Autodesk Fusion 360 part; units mm, degrees
note: some values were not read from the file. Set by a fixed rule: which face or edge a step refers to.
(part 6 of 13)
sketch "Sketch1" plane through (0, 0, 0) normal (0, 0, 1) x (1, 0, 0)
  line L0 (0, 0) -> (25, 0)
  line L1 (25, 0) -> (25, 103)
  line L2 (25, 103) -> (0, 103)
  line L3 (0, 103) -> (0, 0)
  line L4 (0, 0) -> (2.25, 0)
  line L5 (0, 5) -> (25, 5)
  line L6 (0, 98) -> (25, 98)
  line L7 (0, 98) -> (7, 98)
  line L8 (7, 98) -> (7, 103)
  line L9 (7, 103) -> (0, 103)
  line L10 (0, 103) -> (0, 98)
  line L11 (7, 5) -> (0, 5)
  line L12 (0, 5) -> (0, 0)
  line L13 (0, 0) -> (7, 0)
  line L14 (7, 0) -> (7, 5)
  line L15 (10, 5) -> (17, 5)
  line L16 (17, 5) -> (17, 0)
  line L17 (17, 0) -> (10, 0)
  line L18 (10, 0) -> (10, 5)
  line L19 (10, 103) -> (17, 103)
  line L20 (17, 103) -> (17, 98)
  line L21 (17, 98) -> (10, 98)
  line L22 (10, 98) -> (10, 103)
  point P0 (25, 51.5)
  point P1 (25, 51.5)
  dimension "d1" = 25
  dimension "d2" = 103
  constraint horizontal L0
  constraint vertical L1
  constraint horizontal L2
  constraint vertical L3
  constraint coincident L0.start L3.end
  constraint coincident L0 L4.end
  constraint coincident L3 L5.start
  constraint coincident L1 L5.end
  constraint perpendicular L1 L5
  constraint coincident L3 L6.start
  constraint coincident L1 L6.end
  constraint perpendicular L1 L6
  constraint midpoint L1 P1
  constraint coincident P1 P0
  constraint horizontal L7
  constraint vertical L8
  constraint horizontal L9
  constraint vertical L10
  constraint horizontal L11
  constraint vertical L12
  constraint horizontal L13
  constraint vertical L14
  constraint coincident L5 L11.start
  constraint horizontal L15
  constraint vertical L16
  constraint horizontal L17
  constraint vertical L18
  constraint coincident L0 L16.end
  constraint coincident L5 L15.start
  constraint horizontal L19
  constraint vertical L20
  constraint horizontal L21
  constraint vertical L22
  constraint coincident L6 L20.end
  constraint coincident L2 L19.start
  measures "d1" distance of L0.start L0.end
  measures "d2" distance of L0.start L2.end
extrude "Extrude1" add sketch "Sketch1" along normal blind 2.5 contours L0 L3 L4 L5 L11 L12 L13 L14 | L1 L3 L5 L6 L7 L11 L15 L21 | L2 L3 L6 L7 L8 L9 L10 | L0 L5 L15 L16 L17 L18 | L2 L6 L19 L20 L21 L22 makes body 1
copy_body "CopyPasteBodies1" bodies 1 makes body 2
move_body "Move1" bodies 2 to x (1, 0, 0) y (0, 1, 0) z (0, 0, 1) at (37, 0, 0)
copy_body "Body->Comp1" bodies 1 removing the originals makes body 3 in component "Component"
copy_body "Body->Comp2" bodies 2 removing the originals makes body 4 in component "Component'"
component "Component" placed x (1, 0, 0) y (0, 1, 0) z (0, 0, 1) at (0, 0, 0)
component "Component'" placed x (1, 0, 0) y (0, 1, 0) z (0, 0, 1) at (0, 0, 0)

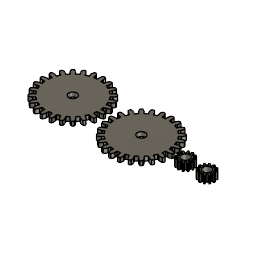
design "card-shuffler-middle-gears"
part number: 2026-08-17-02-18-25-515
part number: 2026-08-17-02-37-57-610
part number: 2026-08-17-02-39-26-180
Autodesk Fusion 360 part; units mm, degrees
sketch "Sketch1" plane through (0, 0, 0) normal (0, 0, 1) x (1, 0, 0) in component "Component"
  spline S0 degree 5 poles (4.55639, -0.625578) (4.556431, -0.625583) (4.556519, -0.625594) (4.556664, -0.625612) (4.556887, -0.625638) (4.557214, -0.625675) (4.557589, -0.625717) (4.558012, -0.625763) (4.558483, -0.625812) (4.559001, -0.625865) (4.559566, -0.625921) (4.560177, -0.62598) (4.560835, -0.62604) (4.561539, -0.626103) (4.562289, -0.626167) (4.563084, -0.626233) (4.563925, -0.626299) (4.564811, -0.626366) (4.565742, -0.626434) (4.566718, -0.626502) (4.567738, -0.62657) (4.568802, -0.626637) (4.569909, -0.626704) (4.571061, -0.626769) (4.572255, -0.626834) (4.573493, -0.626896) (4.574774, -0.626957) (4.576097, -0.627016) (4.577463, -0.627072) (4.578871, -0.627126) (4.580321, -0.627176) (4.581812, -0.627224) (4.583345, -0.627268) (4.584919, -0.627308) (4.586534, -0.627345) (4.58819, -0.627377) (4.589886, -0.627405) (4.591623, -0.627428) (4.5934, -0.627446) (4.595217, -0.627459) (4.597073, -0.627467) (4.598968, -0.627469) (4.600903, -0.627465) (4.602877, -0.627456) (4.60489, -0.627439) (4.606941, -0.627417) (4.60903, -0.627387) (4.611158, -0.627351) (4.613323, -0.627308) (4.615527, -0.627257) (4.617767, -0.627198) (4.620045, -0.627132) (4.62236, -0.627058) (4.624712, -0.626975) (4.6271, -0.626884) (4.629525, -0.626785) (4.631986, -0.626676) (4.634484, -0.626559) (4.637017, -0.626432) (4.639585, -0.626296) (4.642189, -0.626151) (4.644828, -0.625996) (4.647503, -0.62583) (4.650212, -0.625655) (4.652956, -0.625469) (4.655734, -0.625273) (4.658546, -0.625066) (4.661393, -0.624848) (4.664273, -0.624619) (4.667187, -0.624379) (4.670135, -0.624128) (4.673116, -0.623865) (4.67613, -0.62359) (4.679177, -0.623304) (4.682256, -0.623005) (4.685368, -0.622694) (4.688513, -0.622371) (4.691689, -0.622035) (4.694898, -0.621687) (4.698138, -0.621325) (4.70141, -0.620951) (4.704714, -0.620563) (4.708048, -0.620163) (4.711414, -0.619748) (4.714811, -0.61932) (4.718238, -0.618879) (4.721696, -0.618423) (4.725184, -0.617953) (4.728702, -0.61747) (4.732251, -0.616971) (4.735829, -0.616459) (4.739437, -0.615931) (4.743074, -0.615389) (4.74674, -0.614832) (4.750436, -0.61426) (4.754161, -0.613673) (4.757914, -0.613071) (4.761696, -0.612453) (4.765506, -0.611819) (4.769345, -0.61117) (4.773212, -0.610505) (4.777106, -0.609824) (4.781029, -0.609127) (4.784979, -0.608414) (4.788956, -0.607684) (4.792961, -0.606938) (4.796992, -0.606176) (4.801051, -0.605396) (4.805136, -0.6046) (4.809248, -0.603787) (4.813386, -0.602957) (4.817551, -0.60211) (4.821742, -0.601246) (4.825958, -0.600364) (4.830201, -0.599464) (4.834469, -0.598547) (4.838762, -0.597613) (4.843081, -0.59666) (4.847425, -0.59569) (4.851793, -0.594701) (4.856187, -0.593695) (4.860605, -0.59267) (4.865048, -0.591627) (4.869515, -0.590565) (4.874006, -0.589485) (4.878521, -0.588386) (4.88306, -0.587269) (4.887623, -0.586132) (4.892209, -0.584977) (4.896819, -0.583802) (4.901452, -0.582609) (4.906108, -0.581396) (4.910787, -0.580163) (4.915489, -0.578912) (4.920213, -0.577641) (4.92496, -0.57635) (4.929729, -0.57504) (4.93452, -0.573709) (4.939334, -0.572359) (4.944169, -0.570989) (4.949026, -0.569599) (4.953904, -0.568189) (4.958804, -0.566758) (4.963725, -0.565307) (4.968668, -0.563836) (4.973631, -0.562344) (4.978615, -0.560832) (4.98362, -0.559299) (4.988645, -0.557746) (4.993691, -0.556171) (4.998756, -0.554576) (5.003842, -0.55296) (5.008948, -0.551323) (5.014074, -0.549664) (5.01922, -0.547985) (5.024384, -0.546284) (5.029569, -0.544562) (5.034772, -0.542818) (5.039995, -0.541053) (5.045236, -0.539267) (5.050497, -0.537458) (5.055776, -0.535628) (5.061073, -0.533777) (5.066389, -0.531903) (5.071723, -0.530008) (5.077076, -0.528091) (5.082446, -0.526151) (5.087834, -0.52419) (5.093239, -0.522206) (5.098663, -0.5202) (5.104103, -0.518172) (5.109561, -0.516122) (5.115036, -0.514049) (5.120528, -0.511953) (5.126037, -0.509835) (5.131563, -0.507695) (5.137105, -0.505532) (5.142663, -0.503346) (5.148238, -0.501137) (5.153829, -0.498906) (5.159436, -0.496651) (5.165059, -0.494374) (5.170698, -0.492073) (5.176352, -0.48975) (5.182022, -0.487404) (5.187708, -0.485034) (5.193408, -0.482641) (5.199124, -0.480225) (5.204854, -0.477785) (5.210599, -0.475322) (5.21636, -0.472836) (5.222134, -0.470326) (5.227923, -0.467793) (5.233727, -0.465236) (5.239544, -0.462655) (5.245376, -0.460051) (5.251221, -0.457423) (5.257081, -0.454771) (5.262954, -0.452096) (5.26884, -0.449396) (5.27474, -0.446673) (5.280653, -0.443925) (5.28658, -0.441154) (5.292519, -0.438359) (5.298471, -0.435539) (5.304436, -0.432696) (5.310414, -0.429828) (5.316404, -0.426936) (5.322407, -0.42402) (5.328422, -0.421079) (5.334448, -0.418115) (5.340487, -0.415125) (5.346538, -0.412112) (5.352601, -0.409074) (5.358675, -0.406011) (5.364761, -0.402924) (5.370858, -0.399812) (5.376966, -0.396676) (5.383086, -0.393515) (5.389216, -0.39033) (5.395357, -0.387119) (5.40151, -0.383884) (5.407672, -0.380625) (5.413846, -0.37734) (5.420029, -0.374031) (5.426223, -0.370696) (5.432428, -0.367337) (5.438642, -0.363953) (5.444866, -0.360544) (5.4511, -0.35711) (5.457343, -0.353651) (5.463597, -0.350166) (5.469859, -0.346657) (5.476131, -0.343123) (5.482412, -0.339563) (5.488702, -0.335979) (5.495001, -0.332369) (5.501309, -0.328733) (5.507626, -0.325073) (5.513951, -0.321387) (5.520284, -0.317676) (5.525358, -0.314687) (5.529167, -0.312434) (5.531709, -0.310927) (5.53298, -0.310172) knots 0 0 0 0 0 0 0.00416667 0.00833333 0.0125 0.01666667 0.02083333 0.025 0.02916667 0.03333333 0.0375 0.04166667 0.04583333 0.05 0.05416667 0.05833333 0.0625 0.06666667 0.07083333 0.075 0.07916667 0.08333333 0.0875 0.09166667 0.09583333 0.1 0.10416667 0.10833333 0.1125 0.11666667 0.12083333 0.125 0.12916667 0.13333333 0.1375 0.14166667 0.14583333 0.15 0.15416667 0.15833333 0.1625 0.16666667 0.17083333 0.175 0.17916667 0.18333333 0.1875 0.19166667 0.19583333 0.2 0.20416667 0.20833333 0.2125 0.21666667 0.22083333 0.225 0.22916667 0.23333333 0.2375 0.24166667 0.24583333 0.25 0.25416667 0.25833333 0.2625 0.26666667 0.27083333 0.275 0.27916667 0.28333333 0.2875 0.29166667 0.29583333 0.3 0.30416667 0.30833333 0.3125 0.31666667 0.32083333 0.325 0.32916667 0.33333333 0.3375 0.34166667 0.34583333 0.35 0.35416667 0.35833333 0.3625 0.36666667 0.37083333 0.375 0.37916667 0.38333333 0.3875 0.39166667 0.39583333 0.4 0.40416667 0.40833333 0.4125 0.41666667 0.42083333 0.425 0.42916667 0.43333333 0.4375 0.44166667 0.44583333 0.45 0.45416667 0.45833333 0.4625 0.46666667 0.47083333 0.475 0.47916667 0.48333333 0.4875 0.49166667 0.49583333 0.5 0.50416667 0.50833333 0.5125 0.51666667 0.52083333 0.525 0.52916667 0.53333333 0.5375 0.54166667 0.54583333 0.55 0.55416667 0.55833333 0.5625 0.56666667 0.57083333 0.575 0.57916667 0.58333333 0.5875 0.59166667 0.59583333 0.6 0.60416667 0.60833333 0.6125 0.61666667 0.62083333 0.625 0.62916667 0.63333333 0.6375 0.64166667 0.64583333 0.65 0.65416667 0.65833333 0.6625 0.66666667 0.67083333 0.675 0.67916667 0.68333333 0.6875 0.69166667 0.69583333 0.7 0.70416667 0.70833333 0.7125 0.71666667 0.72083333 0.725 0.72916667 0.73333333 0.7375 0.74166667 0.74583333 0.75 0.75416667 0.75833333 0.7625 0.76666667 0.77083333 0.775 0.77916667 0.78333333 0.7875 0.79166667 0.79583333 0.8 0.80416667 0.80833333 0.8125 0.81666667 0.82083333 0.825 0.82916667 0.83333333 0.8375 0.84166667 0.84583333 0.85 0.85416667 0.85833333 0.8625 0.86666667 0.87083333 0.875 0.87916667 0.88333333 0.8875 0.89166667 0.89583333 0.9 0.90416667 0.90833333 0.9125 0.91666667 0.92083333 0.925 0.92916667 0.93333333 0.9375 0.94166667 0.94583333 0.95 0.95416667 0.95833333 0.9625 0.96666667 0.97083333 0.975 0.97916667 0.98333333 0.9875 0.99166667 0.99583333 1 1 1 1 1 1
  spline S1 degree 5 poles (4.55639, 0.625578) (4.556431, 0.625583) (4.556519, 0.625594) (4.556664, 0.625612) (4.556887, 0.625638) (4.557214, 0.625675) (4.557589, 0.625717) (4.558012, 0.625763) (4.558483, 0.625812) (4.559001, 0.625865) (4.559566, 0.625921) (4.560177, 0.62598) (4.560835, 0.62604) (4.561539, 0.626103) (4.562289, 0.626167) (4.563084, 0.626233) (4.563925, 0.626299) (4.564811, 0.626366) (4.565742, 0.626434) (4.566718, 0.626502) (4.567738, 0.62657) (4.568802, 0.626637) (4.569909, 0.626704) (4.571061, 0.626769) (4.572255, 0.626834) (4.573493, 0.626896) (4.574774, 0.626957) (4.576097, 0.627016) (4.577463, 0.627072) (4.578871, 0.627126) (4.580321, 0.627176) (4.581812, 0.627224) (4.583345, 0.627268) (4.584919, 0.627308) (4.586534, 0.627345) (4.58819, 0.627377) (4.589886, 0.627405) (4.591623, 0.627428) (4.5934, 0.627446) (4.595217, 0.627459) (4.597073, 0.627467) (4.598968, 0.627469) (4.600903, 0.627465) (4.602877, 0.627456) (4.60489, 0.627439) (4.606941, 0.627417) (4.60903, 0.627387) (4.611158, 0.627351) (4.613323, 0.627308) (4.615527, 0.627257) (4.617767, 0.627198) (4.620045, 0.627132) (4.62236, 0.627058) (4.624712, 0.626975) (4.6271, 0.626884) (4.629525, 0.626785) (4.631986, 0.626676) (4.634484, 0.626559) (4.637017, 0.626432) (4.639585, 0.626296) (4.642189, 0.626151) (4.644828, 0.625996) (4.647503, 0.62583) (4.650212, 0.625655) (4.652956, 0.625469) (4.655734, 0.625273) (4.658546, 0.625066) (4.661393, 0.624848) (4.664273, 0.624619) (4.667187, 0.624379) (4.670135, 0.624128) (4.673116, 0.623865) (4.67613, 0.62359) (4.679177, 0.623304) (4.682256, 0.623005) (4.685368, 0.622694) (4.688513, 0.622371) (4.691689, 0.622035) (4.694898, 0.621687) (4.698138, 0.621325) (4.70141, 0.620951) (4.704714, 0.620563) (4.708048, 0.620163) (4.711414, 0.619748) (4.714811, 0.61932) (4.718238, 0.618879) (4.721696, 0.618423) (4.725184, 0.617953) (4.728702, 0.61747) (4.732251, 0.616971) (4.735829, 0.616459) (4.739437, 0.615931) (4.743074, 0.615389) (4.74674, 0.614832) (4.750436, 0.61426) (4.754161, 0.613673) (4.757914, 0.613071) (4.761696, 0.612453) (4.765506, 0.611819) (4.769345, 0.61117) (4.773212, 0.610505) (4.777106, 0.609824) (4.781029, 0.609127) (4.784979, 0.608414) (4.788956, 0.607684) (4.792961, 0.606938) (4.796992, 0.606176) (4.801051, 0.605396) (4.805136, 0.6046) (4.809248, 0.603787) (4.813386, 0.602957) (4.817551, 0.60211) (4.821742, 0.601246) (4.825958, 0.600364) (4.830201, 0.599464) (4.834469, 0.598547) (4.838762, 0.597613) (4.843081, 0.59666) (4.847425, 0.59569) (4.851793, 0.594701) (4.856187, 0.593695) (4.860605, 0.59267) (4.865048, 0.591627) (4.869515, 0.590565) (4.874006, 0.589485) (4.878521, 0.588386) (4.88306, 0.587269) (4.887623, 0.586132) (4.892209, 0.584977) (4.896819, 0.583802) (4.901452, 0.582609) (4.906108, 0.581396) (4.910787, 0.580163) (4.915489, 0.578912) (4.920213, 0.577641) (4.92496, 0.57635) (4.929729, 0.57504) (4.93452, 0.573709) (4.939334, 0.572359) (4.944169, 0.570989) (4.949026, 0.569599) (4.953904, 0.568189) (4.958804, 0.566758) (4.963725, 0.565307) (4.968668, 0.563836) (4.973631, 0.562344) (4.978615, 0.560832) (4.98362, 0.559299) (4.988645, 0.557746) (4.993691, 0.556171) (4.998756, 0.554576) (5.003842, 0.55296) (5.008948, 0.551323) (5.014074, 0.549664) (5.01922, 0.547985) (5.024384, 0.546284) (5.029569, 0.544562) (5.034772, 0.542818) (5.039995, 0.541053) (5.045236, 0.539267) (5.050497, 0.537458) (5.055776, 0.535628) (5.061073, 0.533777) (5.066389, 0.531903) (5.071723, 0.530008) (5.077076, 0.528091) (5.082446, 0.526151) (5.087834, 0.52419) (5.093239, 0.522206) (5.098663, 0.5202) (5.104103, 0.518172) (5.109561, 0.516122) (5.115036, 0.514049) (5.120528, 0.511953) (5.126037, 0.509835) (5.131563, 0.507695) (5.137105, 0.505532) (5.142663, 0.503346) (5.148238, 0.501137) (5.153829, 0.498906) (5.159436, 0.496651) (5.165059, 0.494374) (5.170698, 0.492073) (5.176352, 0.48975) (5.182022, 0.487404) (5.187708, 0.485034) (5.193408, 0.482641) (5.199124, 0.480225) (5.204854, 0.477785) (5.210599, 0.475322) (5.21636, 0.472836) (5.222134, 0.470326) (5.227923, 0.467793) (5.233727, 0.465236) (5.239544, 0.462655) (5.245376, 0.460051) (5.251221, 0.457423) (5.257081, 0.454771) (5.262954, 0.452096) (5.26884, 0.449396) (5.27474, 0.446673) (5.280653, 0.443925) (5.28658, 0.441154) (5.292519, 0.438359) (5.298471, 0.435539) (5.304436, 0.432696) (5.310414, 0.429828) (5.316404, 0.426936) (5.322407, 0.42402) (5.328422, 0.421079) (5.334448, 0.418115) (5.340487, 0.415125) (5.346538, 0.412112) (5.352601, 0.409074) (5.358675, 0.406011) (5.364761, 0.402924) (5.370858, 0.399812) (5.376966, 0.396676) (5.383086, 0.393515) (5.389216, 0.39033) (5.395357, 0.387119) (5.40151, 0.383884) (5.407672, 0.380625) (5.413846, 0.37734) (5.420029, 0.374031) (5.426223, 0.370696) (5.432428, 0.367337) (5.438642, 0.363953) (5.444866, 0.360544) (5.4511, 0.35711) (5.457343, 0.353651) (5.463597, 0.350166) (5.469859, 0.346657) (5.476131, 0.343123) (5.482412, 0.339563) (5.488702, 0.335979) (5.495001, 0.332369) (5.501309, 0.328733) (5.507626, 0.325073) (5.513951, 0.321387) (5.520284, 0.317676) (5.525358, 0.314687) (5.529167, 0.312434) (5.531709, 0.310927) (5.53298, 0.310172) knots 0 0 0 0 0 0 0.00416667 0.00833333 0.0125 0.01666667 0.02083333 0.025 0.02916667 0.03333333 0.0375 0.04166667 0.04583333 0.05 0.05416667 0.05833333 0.0625 0.06666667 0.07083333 0.075 0.07916667 0.08333333 0.0875 0.09166667 0.09583333 0.1 0.10416667 0.10833333 0.1125 0.11666667 0.12083333 0.125 0.12916667 0.13333333 0.1375 0.14166667 0.14583333 0.15 0.15416667 0.15833333 0.1625 0.16666667 0.17083333 0.175 0.17916667 0.18333333 0.1875 0.19166667 0.19583333 0.2 0.20416667 0.20833333 0.2125 0.21666667 0.22083333 0.225 0.22916667 0.23333333 0.2375 0.24166667 0.24583333 0.25 0.25416667 0.25833333 0.2625 0.26666667 0.27083333 0.275 0.27916667 0.28333333 0.2875 0.29166667 0.29583333 0.3 0.30416667 0.30833333 0.3125 0.31666667 0.32083333 0.325 0.32916667 0.33333333 0.3375 0.34166667 0.34583333 0.35 0.35416667 0.35833333 0.3625 0.36666667 0.37083333 0.375 0.37916667 0.38333333 0.3875 0.39166667 0.39583333 0.4 0.40416667 0.40833333 0.4125 0.41666667 0.42083333 0.425 0.42916667 0.43333333 0.4375 0.44166667 0.44583333 0.45 0.45416667 0.45833333 0.4625 0.46666667 0.47083333 0.475 0.47916667 0.48333333 0.4875 0.49166667 0.49583333 0.5 0.50416667 0.50833333 0.5125 0.51666667 0.52083333 0.525 0.52916667 0.53333333 0.5375 0.54166667 0.54583333 0.55 0.55416667 0.55833333 0.5625 0.56666667 0.57083333 0.575 0.57916667 0.58333333 0.5875 0.59166667 0.59583333 0.6 0.60416667 0.60833333 0.6125 0.61666667 0.62083333 0.625 0.62916667 0.63333333 0.6375 0.64166667 0.64583333 0.65 0.65416667 0.65833333 0.6625 0.66666667 0.67083333 0.675 0.67916667 0.68333333 0.6875 0.69166667 0.69583333 0.7 0.70416667 0.70833333 0.7125 0.71666667 0.72083333 0.725 0.72916667 0.73333333 0.7375 0.74166667 0.74583333 0.75 0.75416667 0.75833333 0.7625 0.76666667 0.77083333 0.775 0.77916667 0.78333333 0.7875 0.79166667 0.79583333 0.8 0.80416667 0.80833333 0.8125 0.81666667 0.82083333 0.825 0.82916667 0.83333333 0.8375 0.84166667 0.84583333 0.85 0.85416667 0.85833333 0.8625 0.86666667 0.87083333 0.875 0.87916667 0.88333333 0.8875 0.89166667 0.89583333 0.9 0.90416667 0.90833333 0.9125 0.91666667 0.92083333 0.925 0.92916667 0.93333333 0.9375 0.94166667 0.94583333 0.95 0.95416667 0.95833333 0.9625 0.96666667 0.97083333 0.975 0.97916667 0.98333333 0.9875 0.99166667 0.99583333 1 1 1 1 1 1
  spline S2 degree 5 poles (4.55596, -0.625523) (4.555978, -0.625525) (4.556012, -0.625529) (4.556063, -0.625536) (4.556132, -0.625545) (4.556218, -0.625556) (4.556287, -0.625564) (4.556338, -0.625571) (4.556373, -0.625575) (4.55639, -0.625578) knots 0 0 0 0 0 0 0.2 0.4 0.6 0.8 1 1 1 1 1 1
  spline S3 degree 5 poles (4.55596, 0.625523) (4.555978, 0.625525) (4.556012, 0.625529) (4.556063, 0.625536) (4.556132, 0.625545) (4.556218, 0.625556) (4.556287, 0.625564) (4.556338, 0.625571) (4.556373, 0.625575) (4.55639, 0.625578) knots 0 0 0 0 0 0 0.2 0.4 0.6 0.8 1 1 1 1 1 1
  line L0 (0, 0) -> (4.55596, -0.625523)
  line L1 (0, 0) -> (4.55596, 0.625523)
  arc A0 (5.53298, -0.310172) -> (5.53298, 0.310172) centre (0, 0) ccw
  point P0 (4.55768, -0.625727)
  point P1 (4.559834, -0.625946)
  point P2 (4.562853, -0.626213)
  point P3 (4.56674, -0.626503)
  point P4 (4.571494, -0.626792)
  point P5 (4.577117, -0.627057)
  point P6 (4.583608, -0.627274)
  point P7 (4.590968, -0.627418)
  point P8 (4.599194, -0.627467)
  point P9 (4.608287, -0.627397)
  point P10 (4.618244, -0.627183)
  point P11 (4.629062, -0.626802)
  point P12 (4.640739, -0.626231)
  point P13 (4.653272, -0.625445)
  point P14 (4.666656, -0.624422)
  point P15 (4.680887, -0.623137)
  point P16 (4.69596, -0.621567)
  point P17 (4.711871, -0.619689)
  point P18 (4.728613, -0.617479)
  point P19 (4.74618, -0.614915)
  point P20 (4.764565, -0.611974)
  point P21 (4.783761, -0.608632)
  point P22 (4.803761, -0.604867)
  point P23 (4.824556, -0.600655)
  point P24 (4.846137, -0.595976)
  point P25 (4.868496, -0.590805)
  point P26 (4.891623, -0.585122)
  point P27 (4.915508, -0.578903)
  point P28 (4.94014, -0.572128)
  point P29 (4.965509, -0.564774)
  point P30 (4.991603, -0.556821)
  point P31 (5.01841, -0.548246)
  point P32 (5.045918, -0.539029)
  point P33 (5.074114, -0.52915)
  point P34 (5.102985, -0.518586)
  point P35 (5.132518, -0.507319)
  point P36 (5.162698, -0.495328)
  point P37 (5.193511, -0.482593)
  point P38 (5.224943, -0.469095)
  point P39 (5.256977, -0.454814)
  point P40 (5.289598, -0.439731)
  point P41 (5.32279, -0.423829)
  point P42 (5.356536, -0.407087)
  point P43 (5.39082, -0.389488)
  point P44 (5.425624, -0.371015)
  point P45 (5.460931, -0.351649)
  point P46 (5.496722, -0.331374)
  point P47 (4.55768, 0.625727)
  point P48 (4.559834, 0.625946)
  point P49 (4.562853, 0.626213)
  point P50 (4.56674, 0.626503)
  point P51 (4.571494, 0.626792)
  point P52 (4.577117, 0.627057)
  point P53 (4.583608, 0.627274)
  point P54 (4.590968, 0.627418)
  point P55 (4.599194, 0.627467)
  point P56 (4.608287, 0.627397)
  point P57 (4.618244, 0.627183)
  point P58 (4.629062, 0.626802)
  point P59 (4.640739, 0.626231)
  point P60 (4.653272, 0.625445)
  point P61 (4.666656, 0.624422)
  point P62 (4.680887, 0.623137)
  point P63 (4.69596, 0.621567)
  point P64 (4.711871, 0.619689)
  point P65 (4.728613, 0.617479)
  point P66 (4.74618, 0.614915)
  point P67 (4.764565, 0.611974)
  point P68 (4.783761, 0.608632)
  point P69 (4.803761, 0.604867)
  point P70 (4.824556, 0.600655)
  point P71 (4.846137, 0.595976)
  point P72 (4.868496, 0.590805)
  point P73 (4.891623, 0.585122)
  point P74 (4.915508, 0.578903)
  point P75 (4.94014, 0.572128)
  point P76 (4.965509, 0.564774)
  point P77 (4.991603, 0.556821)
  point P78 (5.01841, 0.548246)
  point P79 (5.045918, 0.539029)
  point P80 (5.074114, 0.52915)
  point P81 (5.102985, 0.518586)
  point P82 (5.132518, 0.507319)
  point P83 (5.162698, 0.495328)
  point P84 (5.193511, 0.482593)
  point P85 (5.224943, 0.469095)
  point P86 (5.256977, 0.454814)
  point P87 (5.289598, 0.439731)
  point P88 (5.32279, 0.423829)
  point P89 (5.356536, 0.407087)
  point P90 (5.39082, 0.389488)
  point P91 (5.425624, 0.371015)
  point P92 (5.460931, 0.351649)
  point P93 (5.496722, 0.331374)
sketch "Sketch2" plane through (0, 0, 0) normal (0, 0, 1) x (1, 0, 0) in component "Component"
  circle A0 centre (0, 0) radius 3.760417
extrude "Extrude1" add sketch "Sketch2" along normal blind 5 contours A0 picked at (-1.408263, 1.026971) makes body 1 in component "Component"
extrude "Extrude2" add sketch "Sketch1" along normal blind 5 separate body contours S0 S1 L0 L1 A0 picked at (3.037593, 0) makes body 2 in component "Component"
pattern_circular "C-Pattern1" count 12 over 360 about axis through (0, 0, 1.75) along (0, 0, 1) of "Extrude2" makes body 3 at (1.419579, 0.57881, 1.666667) makes body 4 at (0.939987, 1.211054, 1.666667) makes body 5 at (0.208526, 1.518797, 1.666667) makes body 6 at (-0.57881, 1.419579, 1.666667) makes body 7 at (-1.419579, 0.57881, 1.666667) makes body 8 at (-1.518797, 0.208526, 1.666667) makes body 9 at (-1.419579, -0.57881, 1.666667) makes body 10 at (-0.939987, -1.211054, 1.666667) makes body 11 at (-0.208526, -1.518797, 1.666667) makes body 12 at (0.57881, -1.419579, 1.666667) makes body 13 at (1.211054, -0.939987, 1.666667) in component "Component"
combine "Combine1" operation add target body 1 tool bodies 2 3 4 5 6 7 8 9 10 11 12 13 in component "Component"
sketch "Sketch3" plane through (0, 0, 0) normal (0, 0, 1) x (1, 0, 0) in component "Component"
  line L0 (0, 0) -> (51.568365, 0) construction
  line L1 (51.568365, 0) -> (51.568365, 3) construction
  line L2 (51.568365, 3) -> (0, 3) construction
  line L3 (0, 3) -> (0, 0) construction
  constraint perpendicular L0 L1
  constraint parallel L0 L2
  constraint parallel L1 L3
sketch "Sketch1 (2)" plane through (0, 0, 0) normal (0, 0, 1) x (1, 0, 0) in component "Component'"
  spline S0 degree 5 poles (19.838391, -1.410784) (19.83851, -1.410792) (19.838764, -1.410808) (19.839192, -1.410833) (19.839856, -1.410871) (19.840843, -1.410923) (19.841984, -1.410981) (19.84328, -1.411043) (19.844726, -1.411108) (19.84632, -1.411176) (19.848058, -1.411245) (19.849938, -1.411314) (19.851959, -1.411383) (19.854118, -1.411451) (19.856413, -1.411516) (19.858843, -1.411579) (19.861405, -1.411638) (19.864098, -1.411693) (19.86692, -1.411744) (19.869868, -1.411788) (19.872941, -1.411827) (19.876138, -1.411858) (19.879457, -1.411882) (19.882895, -1.411898) (19.886453, -1.411905) (19.890128, -1.411903) (19.893918, -1.411891) (19.897823, -1.411869) (19.90184, -1.411836) (19.905969, -1.411791) (19.910209, -1.411734) (19.914557, -1.411665) (19.919012, -1.411583) (19.923574, -1.411488) (19.928241, -1.411379) (19.933012, -1.411256) (19.937885, -1.411117) (19.942861, -1.410964) (19.947936, -1.410795) (19.953111, -1.410611) (19.958385, -1.410409) (19.963755, -1.410191) (19.969222, -1.409956) (19.974784, -1.409704) (19.98044, -1.409433) (19.98619, -1.409145) (19.992032, -1.408837) (19.997965, -1.408511) (20.003989, -1.408165) (20.010102, -1.4078) (20.016304, -1.407415) (20.022593, -1.407009) (20.02897, -1.406583) (20.035433, -1.406137) (20.041981, -1.405668) (20.048613, -1.405179) (20.05533, -1.404668) (20.062129, -1.404134) (20.06901, -1.403579) (20.075973, -1.403) (20.083016, -1.402399) (20.090139, -1.401775) (20.097341, -1.401127) (20.104622, -1.400456) (20.111981, -1.399761) (20.119417, -1.399041) (20.126929, -1.398298) (20.134516, -1.397529) (20.142179, -1.396736) (20.149917, -1.395918) (20.157728, -1.395074) (20.165612, -1.394205) (20.173569, -1.39331) (20.181598, -1.392389) (20.189698, -1.391442) (20.197868, -1.390469) (20.206109, -1.389469) (20.21442, -1.388442) (20.222799, -1.387389) (20.231247, -1.386308) (20.239763, -1.385199) (20.248346, -1.384064) (20.256996, -1.3829) (20.265712, -1.381709) (20.274494, -1.380489) (20.283341, -1.379241) (20.292252, -1.377965) (20.301228, -1.37666) (20.310268, -1.375327) (20.31937, -1.373964) (20.328536, -1.372572) (20.337763, -1.371151) (20.347052, -1.369701) (20.356403, -1.368221) (20.365814, -1.366711) (20.375285, -1.365172) (20.384817, -1.363602) (20.394407, -1.362002) (20.404057, -1.360372) (20.413765, -1.358711) (20.423531, -1.35702) (20.433355, -1.355298) (20.443236, -1.353545) (20.453174, -1.351761) (20.463168, -1.349945) (20.473218, -1.348099) (20.483323, -1.346221) (20.493484, -1.344312) (20.503699, -1.342371) (20.513969, -1.340398) (20.524292, -1.338393) (20.534669, -1.336356) (20.545099, -1.334287) (20.555582, -1.332185) (20.566117, -1.330052) (20.576704, -1.327885) (20.587343, -1.325687) (20.598033, -1.323455) (20.608774, -1.321191) (20.619565, -1.318893) (20.630407, -1.316563) (20.641298, -1.314199) (20.652239, -1.311802) (20.663229, -1.309372) (20.674268, -1.306908) (20.685354, -1.304411) (20.69649, -1.30188) (20.707672, -1.299315) (20.718902, -1.296717) (20.73018, -1.294084) (20.741503, -1.291418) (20.752874, -1.288717) (20.76429, -1.285982) (20.775752, -1.283213) (20.78726, -1.280409) (20.798812, -1.277571) (20.81041, -1.274698) (20.822052, -1.271791) (20.833738, -1.268848) (20.845468, -1.265871) (20.857241, -1.262859) (20.869058, -1.259813) (20.880918, -1.256731) (20.892821, -1.253613) (20.904765, -1.250461) (20.916752, -1.247273) (20.928781, -1.24405) (20.940851, -1.240792) (20.952963, -1.237498) (20.965115, -1.234168) (20.977308, -1.230803) (20.989542, -1.227402) (21.001815, -1.223965) (21.014129, -1.220492) (21.026482, -1.216983) (21.038874, -1.213439) (21.051305, -1.209858) (21.063775, -1.206241) (21.076283, -1.202588) (21.08883, -1.198898) (21.101415, -1.195172) (21.114037, -1.19141) (21.126697, -1.187612) (21.139394, -1.183776) (21.152128, -1.179905) (21.164898, -1.175996) (21.177705, -1.172051) (21.190548, -1.168069) (21.203427, -1.164051) (21.216342, -1.159995) (21.229292, -1.155903) (21.242277, -1.151773) (21.255297, -1.147607) (21.268352, -1.143403) (21.281442, -1.139162) (21.294565, -1.134884) (21.307723, -1.130569) (21.320914, -1.126217) (21.334139, -1.121827) (21.347397, -1.1174) (21.360689, -1.112935) (21.374013, -1.108433) (21.387369, -1.103894) (21.400758, -1.099316) (21.41418, -1.094702) (21.427633, -1.090049) (21.441117, -1.085359) (21.454634, -1.080631) (21.468181, -1.075865) (21.48176, -1.071062) (21.495369, -1.06622) (21.509009, -1.061341) (21.52268, -1.056423) (21.53638, -1.051468) (21.550111, -1.046475) (21.563871, -1.041443) (21.577661, -1.036373) (21.59148, -1.031266) (21.605329, -1.02612) (21.619206, -1.020935) (21.633112, -1.015713) (21.647047, -1.010452) (21.66101, -1.005153) (21.675, -0.999815) (21.689019, -0.994439) (21.703066, -0.989025) (21.71714, -0.983572) (21.731241, -0.97808) (21.74537, -0.97255) (21.759525, -0.966982) (21.773707, -0.961375) (21.787916, -0.955729) (21.802151, -0.950044) (21.816412, -0.944321) (21.830699, -0.938559) (21.845012, -0.932758) (21.859351, -0.926919) (21.873715, -0.921041) (21.888104, -0.915123) (21.902518, -0.909167) (21.916957, -0.903173) (21.93142, -0.897139) (21.945908, -0.891066) (21.96042, -0.884954) (21.974957, -0.878803) (21.989517, -0.872613) (22.004101, -0.866384) (22.018708, -0.860116) (22.033339, -0.853809) (22.047993, -0.847463) (22.062671, -0.841078) (22.077371, -0.834653) (22.092094, -0.828189) (22.106839, -0.821687) (22.121606, -0.815144) (22.136396, -0.808563) (22.151207, -0.801942) (22.16604, -0.795282) (22.180895, -0.788583) (22.195771, -0.781844) (22.210669, -0.775066) (22.222604, -0.769612) (22.231565, -0.765504) (22.237543, -0.762757) (22.240534, -0.761382) knots 0 0 0 0 0 0 0.00416667 0.00833333 0.0125 0.01666667 0.02083333 0.025 0.02916667 0.03333333 0.0375 0.04166667 0.04583333 0.05 0.05416667 0.05833333 0.0625 0.06666667 0.07083333 0.075 0.07916667 0.08333333 0.0875 0.09166667 0.09583333 0.1 0.10416667 0.10833333 0.1125 0.11666667 0.12083333 0.125 0.12916667 0.13333333 0.1375 0.14166667 0.14583333 0.15 0.15416667 0.15833333 0.1625 0.16666667 0.17083333 0.175 0.17916667 0.18333333 0.1875 0.19166667 0.19583333 0.2 0.20416667 0.20833333 0.2125 0.21666667 0.22083333 0.225 0.22916667 0.23333333 0.2375 0.24166667 0.24583333 0.25 0.25416667 0.25833333 0.2625 0.26666667 0.27083333 0.275 0.27916667 0.28333333 0.2875 0.29166667 0.29583333 0.3 0.30416667 0.30833333 0.3125 0.31666667 0.32083333 0.325 0.32916667 0.33333333 0.3375 0.34166667 0.34583333 0.35 0.35416667 0.35833333 0.3625 0.36666667 0.37083333 0.375 0.37916667 0.38333333 0.3875 0.39166667 0.39583333 0.4 0.40416667 0.40833333 0.4125 0.41666667 0.42083333 0.425 0.42916667 0.43333333 0.4375 0.44166667 0.44583333 0.45 0.45416667 0.45833333 0.4625 0.46666667 0.47083333 0.475 0.47916667 0.48333333 0.4875 0.49166667 0.49583333 0.5 0.50416667 0.50833333 0.5125 0.51666667 0.52083333 0.525 0.52916667 0.53333333 0.5375 0.54166667 0.54583333 0.55 0.55416667 0.55833333 0.5625 0.56666667 0.57083333 0.575 0.57916667 0.58333333 0.5875 0.59166667 0.59583333 0.6 0.60416667 0.60833333 0.6125 0.61666667 0.62083333 0.625 0.62916667 0.63333333 0.6375 0.64166667 0.64583333 0.65 0.65416667 0.65833333 0.6625 0.66666667 0.67083333 0.675 0.67916667 0.68333333 0.6875 0.69166667 0.69583333 0.7 0.70416667 0.70833333 0.7125 0.71666667 0.72083333 0.725 0.72916667 0.73333333 0.7375 0.74166667 0.74583333 0.75 0.75416667 0.75833333 0.7625 0.76666667 0.77083333 0.775 0.77916667 0.78333333 0.7875 0.79166667 0.79583333 0.8 0.80416667 0.80833333 0.8125 0.81666667 0.82083333 0.825 0.82916667 0.83333333 0.8375 0.84166667 0.84583333 0.85 0.85416667 0.85833333 0.8625 0.86666667 0.87083333 0.875 0.87916667 0.88333333 0.8875 0.89166667 0.89583333 0.9 0.90416667 0.90833333 0.9125 0.91666667 0.92083333 0.925 0.92916667 0.93333333 0.9375 0.94166667 0.94583333 0.95 0.95416667 0.95833333 0.9625 0.96666667 0.97083333 0.975 0.97916667 0.98333333 0.9875 0.99166667 0.99583333 1 1 1 1 1 1
  spline S1 degree 5 poles (19.838391, 1.410784) (19.83851, 1.410792) (19.838764, 1.410808) (19.839192, 1.410833) (19.839856, 1.410871) (19.840843, 1.410923) (19.841984, 1.410981) (19.84328, 1.411043) (19.844726, 1.411108) (19.84632, 1.411176) (19.848058, 1.411245) (19.849938, 1.411314) (19.851959, 1.411383) (19.854118, 1.411451) (19.856413, 1.411516) (19.858843, 1.411579) (19.861405, 1.411638) (19.864098, 1.411693) (19.86692, 1.411744) (19.869868, 1.411788) (19.872941, 1.411827) (19.876138, 1.411858) (19.879457, 1.411882) (19.882895, 1.411898) (19.886453, 1.411905) (19.890128, 1.411903) (19.893918, 1.411891) (19.897823, 1.411869) (19.90184, 1.411836) (19.905969, 1.411791) (19.910209, 1.411734) (19.914557, 1.411665) (19.919012, 1.411583) (19.923574, 1.411488) (19.928241, 1.411379) (19.933012, 1.411256) (19.937885, 1.411117) (19.942861, 1.410964) (19.947936, 1.410795) (19.953111, 1.410611) (19.958385, 1.410409) (19.963755, 1.410191) (19.969222, 1.409956) (19.974784, 1.409704) (19.98044, 1.409433) (19.98619, 1.409145) (19.992032, 1.408837) (19.997965, 1.408511) (20.003989, 1.408165) (20.010102, 1.4078) (20.016304, 1.407415) (20.022593, 1.407009) (20.02897, 1.406583) (20.035433, 1.406137) (20.041981, 1.405668) (20.048613, 1.405179) (20.05533, 1.404668) (20.062129, 1.404134) (20.06901, 1.403579) (20.075973, 1.403) (20.083016, 1.402399) (20.090139, 1.401775) (20.097341, 1.401127) (20.104622, 1.400456) (20.111981, 1.399761) (20.119417, 1.399041) (20.126929, 1.398298) (20.134516, 1.397529) (20.142179, 1.396736) (20.149917, 1.395918) (20.157728, 1.395074) (20.165612, 1.394205) (20.173569, 1.39331) (20.181598, 1.392389) (20.189698, 1.391442) (20.197868, 1.390469) (20.206109, 1.389469) (20.21442, 1.388442) (20.222799, 1.387389) (20.231247, 1.386308) (20.239763, 1.385199) (20.248346, 1.384064) (20.256996, 1.3829) (20.265712, 1.381709) (20.274494, 1.380489) (20.283341, 1.379241) (20.292252, 1.377965) (20.301228, 1.37666) (20.310268, 1.375327) (20.31937, 1.373964) (20.328536, 1.372572) (20.337763, 1.371151) (20.347052, 1.369701) (20.356403, 1.368221) (20.365814, 1.366711) (20.375285, 1.365172) (20.384817, 1.363602) (20.394407, 1.362002) (20.404057, 1.360372) (20.413765, 1.358711) (20.423531, 1.35702) (20.433355, 1.355298) (20.443236, 1.353545) (20.453174, 1.351761) (20.463168, 1.349945) (20.473218, 1.348099) (20.483323, 1.346221) (20.493484, 1.344312) (20.503699, 1.342371) (20.513969, 1.340398) (20.524292, 1.338393) (20.534669, 1.336356) (20.545099, 1.334287) (20.555582, 1.332185) (20.566117, 1.330052) (20.576704, 1.327885) (20.587343, 1.325687) (20.598033, 1.323455) (20.608774, 1.321191) (20.619565, 1.318893) (20.630407, 1.316563) (20.641298, 1.314199) (20.652239, 1.311802) (20.663229, 1.309372) (20.674268, 1.306908) (20.685354, 1.304411) (20.69649, 1.30188) (20.707672, 1.299315) (20.718902, 1.296717) (20.73018, 1.294084) (20.741503, 1.291418) (20.752874, 1.288717) (20.76429, 1.285982) (20.775752, 1.283213) (20.78726, 1.280409) (20.798812, 1.277571) (20.81041, 1.274698) (20.822052, 1.271791) (20.833738, 1.268848) (20.845468, 1.265871) (20.857241, 1.262859) (20.869058, 1.259813) (20.880918, 1.256731) (20.892821, 1.253613) (20.904765, 1.250461) (20.916752, 1.247273) (20.928781, 1.24405) (20.940851, 1.240792) (20.952963, 1.237498) (20.965115, 1.234168) (20.977308, 1.230803) (20.989542, 1.227402) (21.001815, 1.223965) (21.014129, 1.220492) (21.026482, 1.216983) (21.038874, 1.213439) (21.051305, 1.209858) (21.063775, 1.206241) (21.076283, 1.202588) (21.08883, 1.198898) (21.101415, 1.195172) (21.114037, 1.19141) (21.126697, 1.187612) (21.139394, 1.183776) (21.152128, 1.179905) (21.164898, 1.175996) (21.177705, 1.172051) (21.190548, 1.168069) (21.203427, 1.164051) (21.216342, 1.159995) (21.229292, 1.155903) (21.242277, 1.151773) (21.255297, 1.147607) (21.268352, 1.143403) (21.281442, 1.139162) (21.294565, 1.134884) (21.307723, 1.130569) (21.320914, 1.126217) (21.334139, 1.121827) (21.347397, 1.1174) (21.360689, 1.112935) (21.374013, 1.108433) (21.387369, 1.103894) (21.400758, 1.099316) (21.41418, 1.094702) (21.427633, 1.090049) (21.441117, 1.085359) (21.454634, 1.080631) (21.468181, 1.075865) (21.48176, 1.071062) (21.495369, 1.06622) (21.509009, 1.061341) (21.52268, 1.056423) (21.53638, 1.051468) (21.550111, 1.046475) (21.563871, 1.041443) (21.577661, 1.036373) (21.59148, 1.031266) (21.605329, 1.02612) (21.619206, 1.020935) (21.633112, 1.015713) (21.647047, 1.010452) (21.66101, 1.005153) (21.675, 0.999815) (21.689019, 0.994439) (21.703066, 0.989025) (21.71714, 0.983572) (21.731241, 0.97808) (21.74537, 0.97255) (21.759525, 0.966982) (21.773707, 0.961375) (21.787916, 0.955729) (21.802151, 0.950044) (21.816412, 0.944321) (21.830699, 0.938559) (21.845012, 0.932758) (21.859351, 0.926919) (21.873715, 0.921041) (21.888104, 0.915123) (21.902518, 0.909167) (21.916957, 0.903173) (21.93142, 0.897139) (21.945908, 0.891066) (21.96042, 0.884954) (21.974957, 0.878803) (21.989517, 0.872613) (22.004101, 0.866384) (22.018708, 0.860116) (22.033339, 0.853809) (22.047993, 0.847463) (22.062671, 0.841078) (22.077371, 0.834653) (22.092094, 0.828189) (22.106839, 0.821687) (22.121606, 0.815144) (22.136396, 0.808563) (22.151207, 0.801942) (22.16604, 0.795282) (22.180895, 0.788583) (22.195771, 0.781844) (22.210669, 0.775066) (22.222604, 0.769612) (22.231565, 0.765504) (22.237543, 0.762757) (22.240534, 0.761382) knots 0 0 0 0 0 0 0.00416667 0.00833333 0.0125 0.01666667 0.02083333 0.025 0.02916667 0.03333333 0.0375 0.04166667 0.04583333 0.05 0.05416667 0.05833333 0.0625 0.06666667 0.07083333 0.075 0.07916667 0.08333333 0.0875 0.09166667 0.09583333 0.1 0.10416667 0.10833333 0.1125 0.11666667 0.12083333 0.125 0.12916667 0.13333333 0.1375 0.14166667 0.14583333 0.15 0.15416667 0.15833333 0.1625 0.16666667 0.17083333 0.175 0.17916667 0.18333333 0.1875 0.19166667 0.19583333 0.2 0.20416667 0.20833333 0.2125 0.21666667 0.22083333 0.225 0.22916667 0.23333333 0.2375 0.24166667 0.24583333 0.25 0.25416667 0.25833333 0.2625 0.26666667 0.27083333 0.275 0.27916667 0.28333333 0.2875 0.29166667 0.29583333 0.3 0.30416667 0.30833333 0.3125 0.31666667 0.32083333 0.325 0.32916667 0.33333333 0.3375 0.34166667 0.34583333 0.35 0.35416667 0.35833333 0.3625 0.36666667 0.37083333 0.375 0.37916667 0.38333333 0.3875 0.39166667 0.39583333 0.4 0.40416667 0.40833333 0.4125 0.41666667 0.42083333 0.425 0.42916667 0.43333333 0.4375 0.44166667 0.44583333 0.45 0.45416667 0.45833333 0.4625 0.46666667 0.47083333 0.475 0.47916667 0.48333333 0.4875 0.49166667 0.49583333 0.5 0.50416667 0.50833333 0.5125 0.51666667 0.52083333 0.525 0.52916667 0.53333333 0.5375 0.54166667 0.54583333 0.55 0.55416667 0.55833333 0.5625 0.56666667 0.57083333 0.575 0.57916667 0.58333333 0.5875 0.59166667 0.59583333 0.6 0.60416667 0.60833333 0.6125 0.61666667 0.62083333 0.625 0.62916667 0.63333333 0.6375 0.64166667 0.64583333 0.65 0.65416667 0.65833333 0.6625 0.66666667 0.67083333 0.675 0.67916667 0.68333333 0.6875 0.69166667 0.69583333 0.7 0.70416667 0.70833333 0.7125 0.71666667 0.72083333 0.725 0.72916667 0.73333333 0.7375 0.74166667 0.74583333 0.75 0.75416667 0.75833333 0.7625 0.76666667 0.77083333 0.775 0.77916667 0.78333333 0.7875 0.79166667 0.79583333 0.8 0.80416667 0.80833333 0.8125 0.81666667 0.82083333 0.825 0.82916667 0.83333333 0.8375 0.84166667 0.84583333 0.85 0.85416667 0.85833333 0.8625 0.86666667 0.87083333 0.875 0.87916667 0.88333333 0.8875 0.89166667 0.89583333 0.9 0.90416667 0.90833333 0.9125 0.91666667 0.92083333 0.925 0.92916667 0.93333333 0.9375 0.94166667 0.94583333 0.95 0.95416667 0.95833333 0.9625 0.96666667 0.97083333 0.975 0.97916667 0.98333333 0.9875 0.99166667 0.99583333 1 1 1 1 1 1
  spline S2 degree 5 poles (19.837349, -1.410717) (19.837391, -1.41072) (19.837474, -1.410725) (19.837599, -1.410733) (19.837766, -1.410744) (19.837974, -1.410758) (19.838141, -1.410768) (19.838266, -1.410776) (19.838349, -1.410782) (19.838391, -1.410784) knots 0 0 0 0 0 0 0.2 0.4 0.6 0.8 1 1 1 1 1 1
  spline S3 degree 5 poles (19.837349, 1.410717) (19.837391, 1.41072) (19.837474, 1.410725) (19.837599, 1.410733) (19.837766, 1.410744) (19.837974, 1.410758) (19.838141, 1.410768) (19.838266, 1.410776) (19.838349, 1.410782) (19.838391, 1.410784) knots 0 0 0 0 0 0 0.2 0.4 0.6 0.8 1 1 1 1 1 1
  line L0 (0, 0) -> (19.837349, -1.410717)
  line L1 (0, 0) -> (19.837349, 1.410717)
  arc A0 (22.240534, -0.761382) -> (22.240534, 0.761382) centre (0, 0) ccw
  point P0 (19.841518, -1.410957)
  point P1 (19.846734, -1.411192)
  point P2 (19.854038, -1.411447)
  point P3 (19.863432, -1.411679)
  point P4 (19.874916, -1.411845)
  point P5 (19.888489, -1.411903)
  point P6 (19.90415, -1.411809)
  point P7 (19.921897, -1.411522)
  point P8 (19.941728, -1.410997)
  point P9 (19.963639, -1.410193)
  point P10 (19.987626, -1.409067)
  point P11 (20.013686, -1.407576)
  point P12 (20.041812, -1.405677)
  point P13 (20.072, -1.403328)
  point P14 (20.104242, -1.400487)
  point P15 (20.138531, -1.397112)
  point P16 (20.17486, -1.393159)
  point P17 (20.213219, -1.388587)
  point P18 (20.253601, -1.383354)
  point P19 (20.295995, -1.377419)
  point P20 (20.340392, -1.370738)
  point P21 (20.386778, -1.363271)
  point P22 (20.435145, -1.354977)
  point P23 (20.485478, -1.345813)
  point P24 (20.537764, -1.335739)
  point P25 (20.591992, -1.324713)
  point P26 (20.648145, -1.312696)
  point P27 (20.70621, -1.299646)
  point P28 (20.76617, -1.285523)
  point P29 (20.828011, -1.270287)
  point P30 (20.891714, -1.253898)
  point P31 (20.957263, -1.236316)
  point P32 (21.024639, -1.217502)
  point P33 (21.093825, -1.197416)
  point P34 (21.1648, -1.17602)
  point P35 (21.237546, -1.153274)
  point P36 (21.312041, -1.129141)
  point P37 (21.388265, -1.103582)
  point P38 (21.466195, -1.076559)
  point P39 (21.545811, -1.048034)
  point P40 (21.627089, -1.017971)
  point P41 (21.710005, -0.986333)
  point P42 (21.794536, -0.953082)
  point P43 (21.880658, -0.918182)
  point P44 (21.968344, -0.881598)
  point P45 (22.05757, -0.843293)
  point P46 (22.148309, -0.803233)
  point P47 (19.841518, 1.410957)
  point P48 (19.846734, 1.411192)
  point P49 (19.854038, 1.411447)
  point P50 (19.863432, 1.411679)
  point P51 (19.874916, 1.411845)
  point P52 (19.888489, 1.411903)
  point P53 (19.90415, 1.411809)
  point P54 (19.921897, 1.411522)
  point P55 (19.941728, 1.410997)
  point P56 (19.963639, 1.410193)
  point P57 (19.987626, 1.409067)
  point P58 (20.013686, 1.407576)
  point P59 (20.041812, 1.405677)
  point P60 (20.072, 1.403328)
  point P61 (20.104242, 1.400487)
  point P62 (20.138531, 1.397112)
  point P63 (20.17486, 1.393159)
  point P64 (20.213219, 1.388587)
  point P65 (20.253601, 1.383354)
  point P66 (20.295995, 1.377419)
  point P67 (20.340392, 1.370738)
  point P68 (20.386778, 1.363271)
  point P69 (20.435145, 1.354977)
  point P70 (20.485478, 1.345813)
  point P71 (20.537764, 1.335739)
  point P72 (20.591992, 1.324713)
  point P73 (20.648145, 1.312696)
  point P74 (20.70621, 1.299646)
  point P75 (20.76617, 1.285523)
  point P76 (20.828011, 1.270287)
  point P77 (20.891714, 1.253898)
  point P78 (20.957263, 1.236316)
  point P79 (21.024639, 1.217502)
  point P80 (21.093825, 1.197416)
  point P81 (21.1648, 1.17602)
  point P82 (21.237546, 1.153274)
  point P83 (21.312041, 1.129141)
  point P84 (21.388265, 1.103582)
  point P85 (21.466195, 1.076559)
  point P86 (21.545811, 1.048034)
  point P87 (21.627089, 1.017971)
  point P88 (21.710005, 0.986333)
  point P89 (21.794536, 0.953082)
  point P90 (21.880658, 0.918182)
  point P91 (21.968344, 0.881598)
  point P92 (22.05757, 0.843293)
  point P93 (22.148309, 0.803233)
sketch "Sketch2 (2)" plane through (0, 0, 0) normal (0, 0, 1) x (1, 0, 0) in component "Component'"
  circle A0 centre (0, 0) radius 18.401984
extrude "Extrude1'" add sketch "Sketch2 (2)" along normal blind 3 separate body contours A0 picked at (6.956077, -5.356629) makes body 14 in component "Component'"
extrude "Extrude2'" add sketch "Sketch1 (2)" along normal blind 3 separate body contours S0 S1 L0 L1 A0 picked at (13.225594, 0) makes body 15 in component "Component'"
pattern_circular "C-Pattern1'" count 24 over 360 about axis through (0, 0, 1.75) along (0, 0, 1) of "Extrude2'" makes body 16 at (6.509184, 1.25728, 1) makes body 17 at (5.961981, 2.89914, 1) makes body 18 at (5.008479, 4.343429, 1) makes body 19 at (3.713657, 5.491719, 2) makes body 20 at (2.165755, 6.265759, 1) makes body 21 at (0.470261, 6.612797, 1) makes body 22 at (-1.25728, 6.509184, 1) makes body 23 at (-2.89914, 5.961981, 1) makes body 24 at (-4.343429, 5.008479, 1) makes body 25 at (-5.961981, 2.89914, 1) makes body 26 at (-6.265759, 2.165755, 2) makes body 27 at (-6.612797, 0.470261, 1) makes body 28 at (-6.509184, -1.25728, 1) makes body 29 at (-5.961981, -2.89914, 1) makes body 30 at (-5.008479, -4.343429, 1) makes body 31 at (-3.713657, -5.491719, 1) makes body 32 at (-2.165755, -6.265759, 1) makes body 33 at (-0.470261, -6.612797, 1) makes body 34 at (1.25728, -6.509184, 1) makes body 35 at (2.89914, -5.961981, 1) makes body 36 at (4.343429, -5.008479, 1) makes body 37 at (5.491719, -3.713657, 1) makes body 38 at (6.265759, -2.165755, 1) in component "Component'"
combine "Combine1'" operation add target body 14 tool bodies 15 16 17 18 19 20 21 22 23 24 25 26 27 28 29 30 31 32 33 34 35 36 37 38 in component "Component'"
sketch "Sketch3 (2)" plane through (0, 0, 0) normal (0, 0, 1) x (1, 0, 0) in component "Component'"
  line L0 (0, 0) -> (67.275882, 0) construction
  line L1 (67.275882, 0) -> (67.275882, 3) construction
  line L2 (67.275882, 3) -> (0, 3) construction
  line L3 (0, 3) -> (0, 0) construction
  constraint perpendicular L0 L1
  constraint parallel L0 L2
  constraint parallel L1 L3